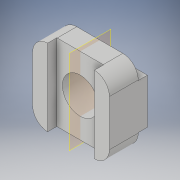
# Autodesk Inventor part: OldhamCouplerMiddle
Saved by Autodesk Inventor 2018 (Build 220112000, 112)
## iProperties
Created: 2017-10-05
Part Number: OldhamCouplerMiddle
Material: Generic
Document SubType Name: Modeling
Designer: Jurjen
Density: 1 g/cm^3
Appearance: Default
Author: Jurjen
Autodesk Inventor part; units mm, degrees
ref_plane "XZ Plane" through (0, 0, 0) normal (0, 1, 0) x (-1, 0, 0)
ref_plane "XY Plane" through (0, 0, 0) normal (0, 0, 1) x (1, 0, 0)
sketch "Sketch1" plane through (0, 0, 0) normal (1, 0, 0) x (0, 1, 0)
  line L0 (-20, 7.5) -> (20, 7.5)
  line L1 (20, 7.5) -> (20, -7.5)
  line L2 (20, -7.5) -> (11.75, -7.5)
  line L3 (11.75, -7.5) -> (11.75, -12.3)
  line L4 (11.75, -12.3) -> (-11.75, -12.3)
  line L5 (-11.75, -12.3) -> (-11.75, -7.5)
  line L6 (-11.75, -7.5) -> (-20, -7.5)
  line L7 (-20, -7.5) -> (-20, 7.5)
  point P0 (0, 0)
  point P1 (0, 7.5)
  point P2 (20, 0)
  point P3 (0, -12.3)
  dimension "d0" = 15
  dimension "d1" = 40
  dimension "d2" = 4.8
  dimension "d3" = 23.5
  constraints: 16 end point, 6 perpendicular, 3 midpoint, 2 point on line, 2 vertical alignment, 1 horizontal, 1 horizontal alignment
  measures "d0" distance of L0.end L1.end
  measures "d1" distance of L0.start L0.end
  measures "d2" distance of L2.end L3.end
  measures "d3" distance of L3.end L4.end
extrude "Extrusion1" add sketch "Sketch1" along normal mid plane 40
sketch "Sketch2" plane through (-20, 20, 7.5) normal (0, 1, 0) x (1, 0, 0)
  line L0 (32.2, 0) -> (7.8, 0)
  line L1 (7.8, 0) -> (7.8, 4.8)
  line L2 (7.8, 4.8) -> (32.2, 4.8)
  line L3 (32.2, 4.8) -> (32.2, 0)
  point P0 (20, 7.5)
  point P1 (40, 0)
  point P2 (20, 4.8)
  dimension "d6" = 24.4
  dimension "d7" = 4.8
  constraints: 8 end point, 2 parallel, 1 horizontal, 1 horizontal alignment, 1 midpoint, 1 perpendicular, 1 vertical alignment
  measures "d6" distance between parallel lines of L1 L3
  measures "d7" distance between parallel lines of L0 L2
extrude "Extrusion2" cut sketch "Sketch2" against normal up to next
fillet "Fillet1" radius 8 4 edges at (20, 20, 0) (-20, 20, 0) (-20, -20, 0) (20, -20, 0)
sketch "Sketch3" plane through (-12, 20, 2.7) normal (0, 0, 1) x (1, 0, 0)
  circle A0 centre (12, -20) radius 9.3
  dimension "d11" = 18.6
  constraints: 1 centre point, 1 coincident
  measures "d11" diameter of A0
extrude "Extrusion3" cut sketch "Sketch3" against normal up to next
body "Solid1"
